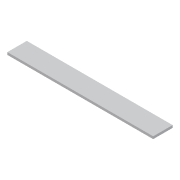
# Autodesk Inventor part: ScaleCompartment_SidePanel
Saved by Autodesk Inventor 2016 (Build 200138000, 138)
## iProperties
Created: 2014-11-25
Part Number: ScaleCompartment_SidePanel
Material: Polycarbonat, klar
Document SubType Name: Modeling
Designer: Gero Hofmann
Density: 1.2 g/cm^3
Appearance: Polycarbonat - klar
Author: Gero Hofmann
Autodesk Inventor part; units mm, degrees
ref_plane "YZ Plane" through (0, 0, 0) normal (1, 0, 0) x (0, 1, 0)
ref_plane "XZ Plane" through (0, 0, 0) normal (0, 1, 0) x (-1, 0, 0)
ref_plane "XY Plane" through (0, 0, 0) normal (0, 0, 1) x (1, 0, 0)
sketch "Skizze1" plane through (0, 0, 0) normal (0, 0, 1) x (1, 0, 0)
  line L0 (-300, -40) -> (300, -40)
  line L1 (300, -40) -> (300, 40)
  line L2 (300, 40) -> (-300, 40)
  line L3 (-300, 40) -> (-300, -40)
  line L4 (-300, -40) -> (300, 40) construction
  line L5 (300, -40) -> (-300, 40) construction
  point P0 (0, 0)
  dimension "d0" = 600
  dimension "d1" = 80
  constraints: 12 end point, 2 midpoint, 2 parallel, 1 horizontal, 1 perpendicular
  measures "d0" distance of L2.end L1.end
  measures "d1" distance of L1.end L0.end
extrude "Extrusion1" add sketch "Skizze1" along normal blind 10
